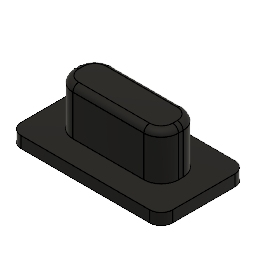
button_select (Autodesk Fusion 360 design; units mm, degrees)
Autodesk Fusion 360 part; units mm, degrees
sketch "Sketch1" plane through (0, 0, 0) normal (0, 1, 0) x (1, 0, 0)
  line L0 (4.575, -1.7) -> (-4.575, -1.7)
  line L1 (-4.575, -1.7) -> (-4.575, 1.7)
  line L2 (-4.575, 1.7) -> (4.575, 1.7)
  line L3 (4.575, 1.7) -> (4.575, -1.7)
  line L4 (4.575, -1.7) -> (-4.575, 1.7) construction
  line L5 (-4.575, -1.7) -> (4.575, 1.7) construction
  dimension "d1" = 9.15
  dimension "d2" = 3.4
  measures "d1" distance of L1.end L2.end
  measures "d2" distance of L0.end L1.end
extrude "Extrude1" add sketch "Sketch1" along normal blind 4
sketch "Sketch2" plane through (0, 0, 0) normal (0, -1, 0) x (1, 0, 0)
  line L0 (-4.575, -1.7) -> (4.575, -1.7)
  line L1 (4.575, -1.7) -> (4.575, 1.7)
  line L2 (4.575, 1.7) -> (-4.575, 1.7)
  line L3 (-4.575, 1.7) -> (-4.575, -1.7)
  line L4 (6.575, -3.7) -> (-6.575, -3.7)
  line L5 (-6.575, -3.7) -> (-6.575, 3.7)
  line L6 (-6.575, 3.7) -> (6.575, 3.7)
  line L7 (6.575, 3.7) -> (6.575, -3.7)
  line L8 (6.575, -3.7) -> (-6.575, 3.7) construction
  line L9 (-6.575, -3.7) -> (6.575, 3.7) construction
  dimension "d5" = 13.15
  dimension "d6" = 7.4
  measures "d5" distance of L5.end L6.end
  measures "d6" distance of L4.end L5.end
extrude "Extrude2" add sketch "Sketch2" along normal blind 1 contours L0 L1 L2 L3 | L4 L5 L6 L7
fillet "Fillet1" radius 1.5 4 edges at (4.575, 2, 1.7) (4.575, 2, -1.7) (-4.575, 2, 1.7) (-4.575, 2, -1.7)
fillet "Fillet2" radius 0.5 8 edges at (4.1357, 4, -1.2607) (0, 4, -1.7) (-4.1357, 4, -1.2607) (-4.575, 4, 0) (-4.1357, 4, 1.2607) (0, 4, 1.7) (4.1357, 4, 1.2607) (4.575, 4, 0)
fillet "Fillet3" radius 1 4 edges at (6.575, -0.5, 3.7) (6.575, -0.5, -3.7) (-6.575, -0.5, 3.7) (-6.575, -0.5, -3.7)
sketch "Sketch3" plane through (0, -1, 0) normal (0, -1, 0) x (1, 0, 0)
  arc A0 (-6.575, -2.7) -> (-5.575, -3.7) centre (-5.575, -2.7) ccw
  line L0 (-5.575, -3.7) -> (5.575, -3.7)
  arc A1 (5.575, -3.7) -> (6.575, -2.7) centre (5.575, -2.7) ccw
  line L1 (6.575, -2.7) -> (6.575, 2.7)
  arc A2 (6.575, 2.7) -> (5.575, 3.7) centre (5.575, 2.7) ccw
  line L2 (5.575, 3.7) -> (-5.575, 3.7)
  arc A3 (-5.575, 3.7) -> (-6.575, 2.7) centre (-5.575, 2.7) ccw
  line L3 (-6.575, 2.7) -> (-6.575, -2.7)
  line L4 (1.6, -1.6) -> (-1.6, -1.6)
  line L5 (-1.6, -1.6) -> (-1.6, 1.6)
  line L6 (-1.6, 1.6) -> (1.6, 1.6)
  line L7 (1.6, 1.6) -> (1.6, -1.6)
  line L8 (1.6, -1.6) -> (-1.6, 1.6) construction
  line L9 (-1.6, -1.6) -> (1.6, 1.6) construction
  dimension "d12" = 3.2
  dimension "d13" = 3.2
  measures "d12" distance of L5.end L6.end
  measures "d13" distance of L4.end L5.end
extrude "Extrude3" cut sketch "Sketch3" against normal blind 2.7 contours L4 L5 L6 L7
chamfer "Chamfer1" distance 0.5 angle 45 4 edges at (1.6, -1, 0) (0, -1, -1.6) (0, -1, 1.6) (-1.6, -1, 0)
